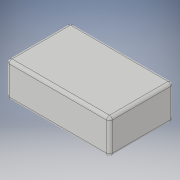
# Autodesk Inventor part: Battery_Model
Saved by Autodesk Inventor 2019 (Build 230136000, 136)
## iProperties
Created: 2019-11-23
Part Number: Battery_Model
Material: Generic
Document SubType Name: Modeling
Designer: Next
Density: 1 g/cm^3
Appearance: Default
Author: Next
Autodesk Inventor part; units mm, degrees
ref_plane "YZ Plane" through (0, 0, 0) normal (1, 0, 0) x (0, 1, 0)
ref_plane "XZ Plane" through (0, 0, 0) normal (0, 1, 0) x (-1, 0, 0)
ref_plane "XY Plane" through (0, 0, 0) normal (0, 0, 1) x (1, 0, 0)
sketch "Sketch1" plane through (0, 0, 0) normal (0, 1, 0) x (-1, 0, 0)
  line L0 (0, 0) -> (-114.3, 0)
  line L1 (-114.3, 0) -> (-114.3, -71.12)
  line L2 (-114.3, -71.12) -> (0, -71.12)
  line L3 (0, -71.12) -> (0, 0)
  dimension "d0" = 114.3
  dimension "d1" = 71.12
  constraints: 8 end point, 2 parallel, 1 horizontal, 1 perpendicular
  measures "d0" distance of L2.end L1.end
  measures "d1" distance of L1.end L0.end
extrude "Extrusion1" add sketch "Sketch1" along normal blind 38.1
fillet "Fillet1" radius 3.175 12 edges at (57.15, 38.1, 0) (114.3, 38.1, -35.56) (57.15, 38.1, -71.12) (0, 38.1, -35.56) (0, 19.05, 0) (114.3, 19.05, 0) (114.3, 19.05, -71.12) (114.3, 0, -35.56) (57.15, 0, -71.12) (57.15, 0, 0) (0, 0, -35.56) (0, 19.05, -71.12)
body "Solid1"
